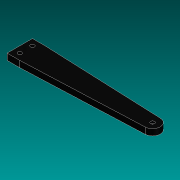
# Autodesk Inventor part: 胴体_サブフレーム_1_12
Saved by Autodesk Inventor 2016 (Build 200138000, 138)
## iProperties
Created: 2016-05-25
Part Number: 胴体_サブフレーム_1_12
Material: アセタール樹脂、黒
Document SubType Name: Modeling
Designer: hiroaki
Density: 1.425 g/cm^3
Appearance: 滑らか - 黒
Mass: 7.28983 g
Surface Area: 57.2603 cm^2
Volume: 5.11567 cm^3
Author: hiroaki
Autodesk Inventor part; units mm, degrees
ref_plane "YZ Plane" through (0, 0, 0) normal (1, 0, 0) x (0, 1, 0)
ref_plane "XZ Plane" through (0, 0, 0) normal (0, 1, 0) x (-1, 0, 0)
ref_plane "XY Plane" through (0, 0, 0) normal (0, 0, 1) x (1, 0, 0)
sketch "スケッチ1" plane through (0, 0, 0) normal (0, 0, 1) x (1, 0, 0)
  circle A0 centre (0, 5) radius 1.55
  circle A1 centre (0, -5) radius 1.55
  line L0 (0, 5) -> (0, -5) construction
  line L1 (0, 0) -> (100, 0) construction
  circle A2 centre (100, 0) radius 1.55
  line L2 (-5, 10) -> (-5, -10)
  line L3 (-5, -10) -> (5, -10)
  line L4 (5, -10) -> (100.2521, -5.9947)
  line L5 (-5, 10) -> (5, 10)
  line L6 (5, 10) -> (100.2521, 5.9947)
  arc A3 (100.2521, -5.9947) -> (100.2521, 5.9947) centre (100, 0) ccw
  circle A4 centre (0, 5) radius 3 construction
  circle A5 centre (0, 5) radius 5 construction
  line L7 (5, 10) -> (5, -10) construction
  point P0 (-5, 0)
  dimension "d0" = 10
  dimension "d1" = 3.1
  dimension "d2" = 3.1
  dimension "d3" = 100
  dimension "d4" = 6
  dimension "d5" = 6
  dimension "d6" = 2
  constraints: 16 end point, 6 centre point, 5 tangent, 4 coincident, 3 vertical, 2 horizontal, 2 midpoint, 2 point on circle, 1 equal radius, 1 horizontal alignment, 1 perpendicular
  measures "d0" distance of L0.start L0.end
  measures "d1" diameter of A0
  measures "d2" diameter of A2
  measures "d3" distance of L1.start L1.end
  measures "d4" radius of A3
  measures "d5" diameter of A4
  measures "d6" radial gap between concentric circles of A5 A4
extrude "押し出し1" add sketch "スケッチ1" along normal blind 5
sketch "スケッチ2" plane through (0, 0, 0) normal (0, 0, -1) x (-1, 0, 0)
  circle A0 centre (-100, 0) radius 1.55 projected
  arc A1 (-100.2521, 5.9947) -> (-100.2521, -5.9947) centre (-100, 0) ccw projected
  circle A2 centre (-100, 0) radius 4.05
  point P0 (0, 0)
  dimension "d9" = 8.1
  constraints: 1 centre point, 1 coincident
  measures "d9" diameter of A2
extrude "押し出し2" cut sketch "スケッチ2" against normal blind 3
sketch "スケッチ3" plane through (0, 0, 0) normal (0, 0, -1) x (-1, 0, 0)
  circle A0 centre (0, -5) radius 1.55 projected
  circle A1 centre (0, 5) radius 1.55 projected
  line L0 (0, -1.8246) -> (2.75, -3.4123)
  line L1 (2.75, -3.4123) -> (2.75, -6.5877)
  line L2 (2.75, -6.5877) -> (0, -8.1754)
  line L3 (0, -8.1754) -> (-2.75, -6.5877)
  line L4 (-2.75, -6.5877) -> (-2.75, -3.4123)
  line L5 (-2.75, -3.4123) -> (0, -1.8246)
  line L6 (-2.75, 6.5877) -> (0, 8.1754)
  line L7 (0, 8.1754) -> (2.75, 6.5877)
  line L8 (2.75, 6.5877) -> (2.75, 3.4123)
  line L9 (2.75, 3.4123) -> (0, 1.8246)
  line L10 (0, 1.8246) -> (-2.75, 3.4123)
  line L11 (-2.75, 3.4123) -> (-2.75, 6.5877)
  line L12 (0, -8.2332) -> (2.8, -6.6166)
  line L13 (2.8, -6.6166) -> (2.8, -3.3834)
  line L14 (2.8, -3.3834) -> (0, -1.7668)
  line L15 (0, -1.7668) -> (-2.8, -3.3834)
  line L16 (-2.8, -3.3834) -> (-2.8, -6.6166)
  line L17 (-2.8, -6.6166) -> (0, -8.2332)
  line L18 (-2.8, 3.3834) -> (0, 1.7668)
  line L19 (0, 1.7668) -> (2.8, 3.3834)
  line L20 (2.8, 3.3834) -> (2.8, 6.6166)
  line L21 (2.8, 6.6166) -> (0, 8.2332)
  line L22 (0, 8.2332) -> (-2.8, 6.6166)
  line L23 (-2.8, 6.6166) -> (-2.8, 3.3834)
  circle A2 centre (0, -7.1832) radius 1.05
  circle A3 centre (1.8907, -6.0916) radius 1.05
  circle A4 centre (1.8907, -3.9084) radius 1.05
  circle A5 centre (0, -2.8168) radius 1.05
  circle A6 centre (-1.8907, -3.9084) radius 1.05
  circle A7 centre (-1.8907, -6.0916) radius 1.05
  circle A8 centre (0, 2.8168) radius 1.05
  circle A9 centre (1.8907, 3.9084) radius 1.05
  circle A10 centre (1.8907, 6.0916) radius 1.05
  circle A11 centre (0, 7.1832) radius 1.05
  circle A12 centre (-1.8907, 6.0916) radius 1.05
  circle A13 centre (-1.8907, 3.9084) radius 1.05
  point P0 (0, 0)
  point P1 (2.8, -6.6166)
  point P2 (2.8, -3.3834)
  point P3 (0, -1.7668)
  point P4 (-2.8, -3.3834)
  point P5 (-2.8, -6.6166)
  point P6 (2.8, 3.3834)
  point P7 (2.8, 6.6166)
  point P8 (0, 8.2332)
  point P9 (-2.8, 6.6166)
  point P10 (-2.8, 3.3834)
  dimension "d16" = 2.1
  dimension "d15" = 5.5
  dimension "d17" = 0.05
  dimension "d20" = 360
  dimension "d24" = 360
  constraints: 48 end point, 6 vertical alignment, 2 coincident, 2 equal length, 2 vertical, 106 other
  measures "d15" distance between parallel lines of L9 L6
  measures "d17" distance between parallel lines of L17 L3
extrude "押し出し3" cut sketch "スケッチ3" against normal blind 1
sketch "スケッチ4" plane through (0, 0, 0) normal (0, 0, -1) x (-1, 0, 0)
  circle A0 centre (-100, 0) radius 4.05 projected
  line L0 (-100.2521, 5.9947) -> (-5, 10) projected
  arc A1 (-100.2521, 5.9947) -> (-100.2521, -5.9947) centre (-100, 0) ccw projected
  line L1 (-5, -10) -> (-100.2521, -5.9947) projected
  line L2 (-7.8, -6.8796) -> (-94.9345, -3.2157)
  line L3 (-5, -10) -> (-100.2521, -5.9947) projected
  arc A2 (-94.9345, -3.2157) -> (-94.9345, 3.2157) centre (-100, 0) ccw
  line L4 (-94.9345, 3.2157) -> (-7.8, 6.8796)
  line L5 (-7.8, 6.8796) -> (-7.8, -6.8796)
  point P0 (-2.8, 4.4334)
  point P1 (0, 0)
  dimension "d26" = 3
  dimension "d27" = 3
  dimension "d28" = 5
  constraints: 6 end point, 3 parallel, 2 point on circle, 1 centre point, 1 coincident, 1 concentric, 1 vertical
  measures "d26" distance between parallel lines of L1 L2
  measures "d27" distance between parallel lines of L0 L4
  measures "d28" distance from line of point (-2.8, 4.433) L5
extrude "押し出し4" cut sketch "スケッチ4" against normal blind 4 contours L2 A2 L4 L5
fillet "フィレット1" radius 2 4 edges at (7.8, 6.8796, 2) (7.8, -6.8796, 2) (94.9345, 3.2157, 2) (94.9345, -3.2157, 2)
equation "\"d27\" = d26"
